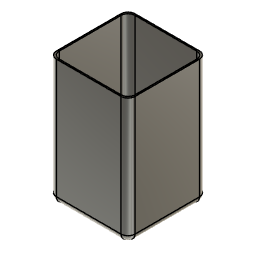
couvre_micro_elgato v1 (Autodesk Fusion 360 design; units mm, degrees)
Autodesk Fusion 360 part; units mm, degrees
sketch "Esquisse1" plane through (0, 0, 0) normal (0, 0, 1) x (1, 0, 0)
  line L0 (0, 0) -> (54, 0)
  line L1 (54, 0) -> (54, 54)
  line L2 (54, 54) -> (0, 54)
  line L3 (0, 54) -> (0, 0)
  line L4 (55, -1) -> (55, 55)
  line L5 (55, 55) -> (-1, 55)
  line L6 (-1, 55) -> (-1, -1)
  line L7 (-1, -1) -> (55, -1)
  line L8 (27, 54) -> (27, 0)
  circle A0 centre (27, 27) radius 5
  dimension "d4" = 54
  dimension "d5" = 54
  dimension "d6" = 1
  dimension "d20" = 10
  constraint horizontal L0
  constraint vertical L1
  constraint horizontal L2
  constraint vertical L3
  constraint coincident L0.start L3.end
  constraint midpoint L2 L8.start
  constraint midpoint L0 L8.end
  constraint midpoint L8 A0.centre
  measures "d4" distance of L0.start L0.end
  measures "d5" distance of L0.start L2.end
  measures "d20" diameter of A0
extrude "Extrusion1" add sketch "Esquisse1" along normal blind 90
extrude "Extrusion2" add sketch "Esquisse1" along normal blind 1 contours L0 L2 L3 L8 A0 | L0 L1 L2 L8 A0 | L8 A0 | L8 A0
fillet "Congé1" radius 5 4 edges at (0, 54, 45.5) (54, 54, 45.5) (54, 0, 45.5) (0, 0, 45.5)
fillet "Congé2" radius 5 8 edges at (52.5355, 52.5355, 1) (54, 27, 1) (52.5355, 1.4645, 1) (27, 0, 1) (1.4645, 1.4645, 1) (0, 27, 1) (1.4645, 52.5355, 1) (27, 54, 1)
fillet "Congé3" radius 5 4 edges at (-1, 55, 45) (55, 55, 45) (55, -1, 45) (-1, -1, 45)
fillet "Congé4" radius 5 8 edges at (55, 27, 0) (53.5355, 53.5355, 0) (27, 55, 0) (0.4645, 53.5355, 0) (-1, 27, 0) (0.4645, 0.4645, 0) (27, -1, 0) (53.5355, 0.4645, 0)
extrude "Extrusion3" cut sketch "Esquisse1" along normal blind 1 contours L8 A0 | L8 A0
equation "base_largeur = 54 mm"
equation "epaisseur = 1 mm"
equation "hauteur = 90 mm"
equation "d4 = base_largeur"
equation "d5 = base_largeur"
equation "d6 = epaisseur"
equation "d7 = hauteur"
equation "d9 = epaisseur"
equation "angle_int = 5 mm"
equation "d13 = angle_int"
equation "d15 = angle_int"
equation "d17 = angle_int"
equation "d19 = angle_int"
equation "d21 = epaisseur"
